Autodesk Inventor part; units mm, degrees
(part 2 of 2)
sketch "Sketch19" plane through (0, 0, 1.5875) normal (0, 0, 1) x (1, 0, 0)
  circle A0 centre (-131.6773, 209.9079) radius 3.5177
  circle A1 centre (-196.794, 254.6594) radius 2.2655
  circle A2 centre (-187.6385, 209.9079) radius 3.5177
  circle A3 centre (-133.294, 368.9594) radius 2.2479
  point P0 (-499.1548, 359.6218)
  point P1 (-499.3886, 356.3852)
  point P2 (-499.1548, 97.7443)
  point P3 (-499.3886, 94.5077)
  point P4 (-499.3886, 159.8698)
  point P5 (-499.1548, 156.6332)
  point P6 (-499.3886, 421.7473)
  point P7 (-499.1548, 418.5107)
sheet face with bend "Face4" sketch "Sketch19" thickness 1.5875 toward (0, 0, -1) bend radius 1.5875 relief tear relief width 1.5875 relief depth 0.7937
bend "Bend3"
extrude "Cut10" cut sketch "Sketch17" against normal blind 1.5875 contours L238 A322 L237 L26 | L26 L237 A323 L238 | L236 A320 L30 E3 L33 L235 L26 | L26 L235 A321 L236 | L234 L33 L233 L26 | L26 L233 A319 L234 | L33 E3 L30 A320 L235 | L234 A318 L233 L33 | A301 L216 A300 L31 E0 L30 | L30 E0 L31 A300 L215 A301 | L232 L33 L231 L26 | L26 L231 A317 L232 | L232 A316 L231 L33 | L230 A314 L32 E2 L33 | L33 E2 L32 A314 L229 A315 L230 | A296 L31 | L31 A296 L211 A297 L212 | A295 L210 A294 L31 E1 L32 | L32 E1 L31 A294 L209 A295 | L247 A333 L248 L37 | L37 L248 A332 L247 | A328 L243 A329 L43 | L43 A329 L244 A328 | A326 L241 A327 L45 | L45 A327 L242 A326 | A197 L112 A196 L51 | L51 A196 L111 A197 | A177 L92 A176 L51 | L51 A176 L91 A177 | A219 L53 | L53 A219 L134 A218 L133 | A221 L53 | L53 A221 L136 A220 L135 | A158 L73 A159 L74 L54 | L54 A158 | A160 L75 A161 L76 L54 | L54 A160 | A203 L118 A202 L52 | L52 A202 L117 A203 | A183 L98 A182 L52 | L52 A182 L97 A183 | A151 L66 A150 L65 | A169 L84 A168 L83 | A171 L86 A170 L85 | A179 L94 A178 L93 | A181 L96 A180 L95 | A189 L104 A188 L103 | A191 L106 A190 L105 | A199 L114 A198 L113 | A201 L116 A200 L115 | A209 L124 A208 L123 | A211 L126 A210 L125 | A229 L144 A228 L143 | A239 L154 A238 L153 | A241 L156 A240 L155 | A259 L174 A258 L173 | A261 L176 A260 L175 | A279 L194 A278 L193 | A281 L196 A280 L195 | A291 L206 A290 L205 | A303 L218 A302 L217 | A305 L220 A304 L219 | A311 L226 A310 L225 | A325 L240 A324 L239 | A331 L246 A330 L245 | A335 L250 A334 L249 | A337 L252 A336 L251 | A339 L254 A338 L253 | A341 L256 A340 L255 | A343 L258 A342 L257 | A345 L260 A344 L259
sheet face with bend "Face5" sketch "Sketch21" thickness 1.5875 toward (0, 0, 1) bend radius 1.5875 relief tear relief width 1.5875 relief depth 0.7937
bend "Bend4"
equation "\"d17\" = Thickness"
equation "\"d65\" = Thickness"
equation "\"BendRadius\" = Thickness"
equation "\"BendReliefWidth\" = Thickness"
equation "\"BendReliefDepth\" = 0.5 * Thickness"
equation "\"CornerReliefSize\" = 4 * Thickness"
equation "\"MinimumRemnant\" = 2 * Thickness"
equation "\"TransitionRadius\" = BendRadius"
equation "\"JacobiRadiusSize\" = Thickness"
equation "\"GapSize\" = Thickness"
equation "\"d2\" = BendRadius"
equation "\"Thickness\" = 1.5875"
body "Solid1"
